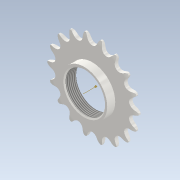
# Autodesk Inventor part: Roller Chain Sprocket1
Saved by Autodesk Inventor 2021 (Build 250183000, 183)
## iProperties
CustomPartVersion: 1
Created: 2021-04-21
Part Number: Roller Chain Sprocket1
Material: Steel
Document SubType Name: Modeling
Designer: maaro
Density: 1 g/cm^3
Appearance: Steel
Author: maaro
Autodesk Inventor part; units mm, degrees
ref_plane "YZ Plane" through (0, 0, 0) normal (1, 0, 0) x (0, 1, 0)
ref_plane "XZ Plane" through (0, 0, 0) normal (0, 1, 0) x (-1, 0, 0)
ref_plane "XY Plane" through (0, 0, 0) normal (0, 0, 1) x (1, 0, 0)
sketch "Theoretical Tooth Profile" plane through (0, 0, 0) normal (0, 0, 1) x (1, 0, 0)
  circle A0 centre (0, 0) radius 36.5682 construction
  line L0 (0, 0) -> (0, 36.5682) construction
  line L1 (0, 0) -> (12.5071, 34.3629) construction
  circle A1 centre (0, 0) radius 39.8226
  arc A2 (-3.07, 34.1407) -> (3.07, 34.1407) centre (0, 36.5682) ccw
  line L2 (0, 36.5682) -> (12.5071, 34.3629) construction
  line L3 (0, 36.5682) -> (4.8634, 40.4137) construction
  line L4 (4.8634, 40.4137) -> (-4.4154, 36.3898) construction
  arc A3 (6.2396, 39.3308) -> (4.7853, 37.2426) centre (10.6852, 34.6841) ccw
  arc A4 (-4.7853, 37.2426) -> (-6.2396, 39.3308) centre (-10.6852, 34.6841) ccw
  line L5 (-10.6852, 34.6841) -> (-4.7853, 37.2426) construction
  arc A5 (-4.4154, 36.3898) -> (-3.07, 34.1407) centre (4.8634, 40.4137) ccw
  line L6 (-4.4154, 36.3898) -> (-4.7853, 37.2426)
  arc A6 (3.07, 34.1407) -> (4.4154, 36.3898) centre (-4.8634, 40.4137) ccw
  line L7 (4.7853, 37.2426) -> (4.4154, 36.3898)
  line L8 (0, 0) -> (6.9151, 39.2176) construction
  point P0 (6.2535, 35.4655)
  dimension "d0" = 73.1364
  dimension "d2" = 20
  dimension "d3" = 3.9137
  dimension "d10" = 128.333
  dimension "d11" = 14.889
  dimension "d12" = 6.2
  dimension "d13" = 10.1137
  dimension "d14" = 10.85
  dimension "d23" = 3.81
  constraints: 18 end point, 15 point on circle, 7 centre point, 3 coincident, 3 point on line, 3 symmetric about line, 3 tangent, 1 equal radius, 1 midpoint, 1 parallel, 1 vertical, 1 other
  measures "d0" diameter of A0
  measures "d2" angle of L1 L0
  measures "d3" radius of A2
  measures "d10" angle of L3 L0
  measures "d11" angle of L4 L3
  measures "d12" distance of L2.start L3.end
  measures "d13" distance of L3.end L4.end
  measures "d14" distance of A3.centre L0.end
  measures "d23" distance from line of L8.end L2
sketch "Tooth Profile" plane through (0, 0, 0) normal (0, 0, 1) x (1, 0, 0)
  arc A0 (-3.6158, 35.0705) -> (3.6158, 35.0705) centre (0, 36.5682) ccw
  arc A1 (6.1028, 39.3522) -> (3.6158, 35.0705) centre (20.8, 27.9526) ccw
  arc A2 (-3.6158, 35.0705) -> (-6.1028, 39.3522) centre (-20.8, 27.9526) ccw
  line L0 (0, 0) -> (0, 36.5682) construction
  line L1 (0, 36.5682) -> (3.6158, 35.0705) construction
  line L2 (0, 36.5682) -> (-3.6158, 35.0705) construction
  circle A3 centre (0, 0) radius 39.8226 projected
  dimension "d44" = 135
  dimension "d45" = 18.6
  dimension "d46" = 3.9137
  constraints: 9 point on circle, 6 end point, 3 centre point, 2 tangent, 1 coincident, 1 equal radius, 1 vertical, 1 other
  measures "d44" angle of L2 L1
  measures "d45" radius of A1
  measures "d46" radius of A0
sketch "Section Profile" plane through (0, 0, 0) normal (1, 0, 0) x (0, 1, 0)
  line L0 (39.8226, 0) -> (-39.8226, 0) projected
  line L1 (26.5514, 1.5345) -> (-26.5514, 1.5345)
  line L2 (-26.5514, 1.5345) -> (-26.5514, -1.5345)
  line L3 (-26.5514, -1.5345) -> (26.5514, -1.5345)
  line L4 (26.5514, -1.5345) -> (26.5514, 1.5345)
  line L5 (26.5514, 1.5345) -> (39.8226, 1.5345) construction
  line L6 (39.8226, 1.5345) -> (39.8226, -1.5345) construction
  line L7 (39.8226, -1.5345) -> (26.5514, -1.5345) construction
  line L8 (26.5514, -1.5345) -> (26.5514, 1.5345)
  arc A0 (39.8226, 0.7725) -> (35.4897, 1.5345) centre (35.4897, -11.1655) ccw
  arc A1 (35.4897, -1.5345) -> (39.8226, -0.7725) centre (35.4897, 11.1655) ccw
  line L9 (35.4897, 1.5345) -> (0, 1.5345)
  line L10 (0, 1.5345) -> (0, -1.5345)
  line L11 (0, -1.5345) -> (35.4897, -1.5345)
  line L12 (0, 1.5345) -> (0, -1.5345)
  line L13 (39.8226, 0.7725) -> (39.8226, -0.7725)
  point P0 (0, 0)
  point P1 (0, 0)
  dimension "d30" = 3.069
  dimension "d31" = 53.1029
  dimension "d32" = 3.069
  dimension "d33" = 0.762
  dimension "d34" = 12.7
  dimension "d43" = 1.5345
  constraints: 26 end point, 7 midpoint, 5 perpendicular, 4 parallel, 4 point on circle, 3 point on line, 3 symmetric about line, 2 centre point, 2 horizontal, 2 tangent, 1 collinear, 1 other
  measures "d30" distance between parallel lines of L7 L5
  measures "d31" distance between parallel lines of L2 L4
  measures "d32" distance between parallel lines of L3 L1
  measures "d33" distance from line of L13.start L5
  measures "d34" radius of A0
  measures "d43" distance between parallel lines of L3 L0
revolve "Shroud" add sketch "Section Profile" angle 360 about axis through (0, 0, 1.5345) along (0, 0, -1) contours L10 L3 L2 L0 | L0 L2 L1 L10
revolve "Strand" add sketch "Section Profile" angle 360 about axis through (0, 0, 1.5345) along (0, 0, -1) contours L13 A1 L11 L4 L0 | L0 L4 L9 A0 L13 | L4 L3 L10 L0 | L0 L10 L1 L4
pattern_of_one "Strand Pattern"
extrude "Theoretical Tooth" cut sketch "Theoretical Tooth Profile" along normal through all both and the other way through all contours A3 L7 A6 A2 A5 L6 A4 A1 picked at (0, 37.3967)
extrude "Tooth" [suppressed]
pattern_circular "Tooth Pattern" count 18 over 360 about axis through (0, 0, -10) along (0, 0, 1) of "Theoretical Tooth"
ref_plane "Timing Plane" through (0, 36.5682, 0) normal (1, 0, 0) x (0, 1, 0)
sketch "Boceto4" plane through (0, 36.5682, 1.5345) normal (0, 0, 1) x (1, 0, 0)
  arc A0 (19.7278, -7.0668) -> (15.685, -4.7327) centre (0, -36.5682) ccw projected
  circle A1 centre (0, -36.5682) radius 20
  dimension "d60" = 40
  constraints: 1 centre point, 1 coincident
  measures "d60" diameter of A1
extrude "Extrusión4" add sketch "Boceto4" along normal blind 7
hole "Agujero1" at (0, 0, -1.5345) direction (0, 0, 1) diameter 34.3762 end through all thread size "M36x1.5" class "6H" standard "ISO Metric profile"
chamfer "Chaflán1" distance 1 angle 45 1 edges at (0, -17.1881, 8.5345)
equation "\"d3\" = 0.5 * da_Dr + da_SC"
equation "\"d12\" = 0.8 * da_Dr"
equation "\"d13\" = 1.3 * da_Dr + da_SC"
equation "\"d14\" = 1.4 * da_Dr"
equation "\"d23\" = da_Ha"
equation "\"d44\" = da_Alfa"
equation "\"d45\" = da_Re"
equation "\"d46\" = da_Ri"
equation "\"d30\" = da_Bf"
equation "\"d31\" = da_Ds"
equation "\"d32\" = da_Bs"
equation "\"d33\" = da_Ba"
equation "\"d34\" = da_Rx"
equation "\"d40\" = da_pt"
equation "\"form_type\" = 0"
equation "\"da_p\" = 12.7"
equation "\"da_Dr\" = 7.75"
equation "\"da_SC\" = 0.03875"
equation "\"da_Ha\" = 3.81"
equation "\"da_pt\" = 13.92"
equation "\"da_Bf\" = 3.069"
equation "\"da_Ba\" = 0.762"
equation "\"da_Rx\" = 12.7"
equation "\"da_Ra\" = 0.508"
equation "\"da_Bs\" = 3.069"
equation "\"da_Ds\" = 53.10288"
equation "\"da_Re\" = 18.6"
equation "\"da_Ri\" = 3.91375"
equation "\"da_Alfa\" = 135deg"
body "Solid1"
